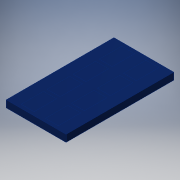
# Autodesk Inventor part: Assembly Plate
Saved by Autodesk Inventor 2019.4 (Build 234330000, 330)
## iProperties
Created: 2021-01-11
Part Number: Assembly Plate
Material: Aluminum, Anodized Blue
Document SubType Name: Modeling
Designer: caleb
Density: 2.7 g/cm^3
Appearance: Anodized - Blue
Author: caleb
Autodesk Inventor part; units mm, degrees
ref_plane "YZ Plane" through (0, 0, 0) normal (1, 0, 0) x (0, 1, 0)
ref_plane "XZ Plane" through (0, 0, 0) normal (0, 1, 0) x (-1, 0, 0)
ref_plane "XY Plane" through (0, 0, 0) normal (0, 0, 1) x (1, 0, 0)
sketch "Sketch1" plane through (0, 0, 0) normal (0, 1, 0) x (-1, 0, 0)
  line L0 (-60, 108) -> (60, 108)
  line L1 (60, 108) -> (60, -108)
  line L2 (60, -108) -> (-60, -108)
  line L3 (-60, -108) -> (-60, 108)
  line L4 (-60, 108) -> (60, -108) construction
  line L5 (60, 108) -> (-60, -108) construction
  point P0 (0, 0)
  dimension "d0" = 120
  dimension "d1" = 216
  constraints: 12 end point, 2 midpoint, 2 parallel, 1 horizontal, 1 perpendicular
  measures "d0" distance of L1.end L2.end
  measures "d1" distance of L0.end L1.end
extrude "Extrusion1" add sketch "Sketch1" along normal blind 14
sketch "Sketch7" plane through (0, 14, 0) normal (0, 1, 0) x (1, 0, 0)
  line L0 (-36.84, -100.8) -> (-11.84, -100.8)
  line L1 (-11.34, -100.3) -> (-11.34, -56.3)
  line L2 (-11.84, -55.8) -> (-36.84, -55.8)
  line L3 (-37.34, -56.3) -> (-37.34, -100.3)
  line L4 (-60, -108) -> (60, -108) projected
  line L5 (-60, 108) -> (-60, -108) projected
  arc A0 (-36.84, -55.8) -> (-37.34, -56.3) centre (-36.84, -56.3) ccw
  arc A1 (-11.34, -56.3) -> (-11.84, -55.8) centre (-11.84, -56.3) ccw
  arc A2 (-11.84, -100.8) -> (-11.34, -100.3) centre (-11.84, -100.3) ccw
  arc A3 (-37.34, -100.3) -> (-36.84, -100.8) centre (-36.84, -100.3) ccw
  arc A4 (-11.84, -48.6) -> (-11.34, -48.1) centre (-11.84, -48.1) ccw
  arc A5 (-37.34, -48.1) -> (-36.84, -48.6) centre (-36.84, -48.1) ccw
  line L6 (-11.34, -48.1) -> (-11.34, -4.1)
  line L7 (-37.34, -4.1) -> (-37.34, -48.1)
  line L8 (-11.84, -3.6) -> (-36.84, -3.6)
  arc A6 (-36.84, -3.6) -> (-37.34, -4.1) centre (-36.84, -4.1) ccw
  arc A7 (-11.34, -4.1) -> (-11.84, -3.6) centre (-11.84, -4.1) ccw
  line L9 (-36.84, -48.6) -> (-11.84, -48.6)
  arc A8 (-11.84, 3.6) -> (-11.34, 4.1) centre (-11.84, 4.1) ccw
  arc A9 (-37.34, 4.1) -> (-36.84, 3.6) centre (-36.84, 4.1) ccw
  line L10 (-11.34, 4.1) -> (-11.34, 48.1)
  line L11 (-37.34, 48.1) -> (-37.34, 4.1)
  line L12 (-11.84, 48.6) -> (-36.84, 48.6)
  arc A10 (-36.84, 48.6) -> (-37.34, 48.1) centre (-36.84, 48.1) ccw
  arc A11 (-11.34, 48.1) -> (-11.84, 48.6) centre (-11.84, 48.1) ccw
  line L13 (-36.84, 3.6) -> (-11.84, 3.6)
  arc A12 (-11.84, 55.8) -> (-11.34, 56.3) centre (-11.84, 56.3) ccw
  arc A13 (-37.34, 56.3) -> (-36.84, 55.8) centre (-36.84, 56.3) ccw
  line L14 (-11.34, 56.3) -> (-11.34, 100.3)
  line L15 (-37.34, 100.3) -> (-37.34, 56.3)
  line L16 (-11.84, 100.8) -> (-36.84, 100.8)
  arc A14 (-36.84, 100.8) -> (-37.34, 100.3) centre (-36.84, 100.3) ccw
  arc A15 (-11.34, 100.3) -> (-11.84, 100.8) centre (-11.84, 100.3) ccw
  line L17 (-36.84, 55.8) -> (-11.84, 55.8)
  arc A16 (36.82, -100.8) -> (37.32, -100.3) centre (36.82, -100.3) ccw
  arc A17 (11.32, -100.3) -> (11.82, -100.8) centre (11.82, -100.3) ccw
  line L18 (37.32, -100.3) -> (37.32, -56.3)
  line L19 (11.32, -56.3) -> (11.32, -100.3)
  line L20 (36.82, -55.8) -> (11.82, -55.8)
  arc A18 (11.82, -55.8) -> (11.32, -56.3) centre (11.82, -56.3) ccw
  arc A19 (37.32, -56.3) -> (36.82, -55.8) centre (36.82, -56.3) ccw
  line L21 (11.82, -100.8) -> (36.82, -100.8)
  arc A20 (36.82, -48.6) -> (37.32, -48.1) centre (36.82, -48.1) ccw
  arc A21 (11.32, -48.1) -> (11.82, -48.6) centre (11.82, -48.1) ccw
  line L22 (37.32, -48.1) -> (37.32, -4.1)
  line L23 (11.32, -4.1) -> (11.32, -48.1)
  line L24 (36.82, -3.6) -> (11.82, -3.6)
  arc A22 (11.82, -3.6) -> (11.32, -4.1) centre (11.82, -4.1) ccw
  arc A23 (37.32, -4.1) -> (36.82, -3.6) centre (36.82, -4.1) ccw
  line L25 (11.82, -48.6) -> (36.82, -48.6)
  arc A24 (36.82, 3.6) -> (37.32, 4.1) centre (36.82, 4.1) ccw
  arc A25 (11.32, 4.1) -> (11.82, 3.6) centre (11.82, 4.1) ccw
  line L26 (37.32, 4.1) -> (37.32, 48.1)
  line L27 (11.32, 48.1) -> (11.32, 4.1)
  line L28 (36.82, 48.6) -> (11.82, 48.6)
  arc A26 (11.82, 48.6) -> (11.32, 48.1) centre (11.82, 48.1) ccw
  arc A27 (37.32, 48.1) -> (36.82, 48.6) centre (36.82, 48.1) ccw
  line L29 (11.82, 3.6) -> (36.82, 3.6)
  arc A28 (36.82, 55.8) -> (37.32, 56.3) centre (36.82, 56.3) ccw
  arc A29 (11.32, 56.3) -> (11.82, 55.8) centre (11.82, 56.3) ccw
  line L30 (37.32, 56.3) -> (37.32, 100.3)
  line L31 (11.32, 100.3) -> (11.32, 56.3)
  line L32 (36.82, 100.8) -> (11.82, 100.8)
  arc A30 (11.82, 100.8) -> (11.32, 100.3) centre (11.82, 100.3) ccw
  arc A31 (37.32, 100.3) -> (36.82, 100.8) centre (36.82, 100.3) ccw
  line L33 (11.82, 55.8) -> (36.82, 55.8)
  point P0 (0, 0)
  point P1 (-37.34, -100.8)
  point P2 (-11.34, -100.8)
  point P3 (-37.34, -55.8)
  point P4 (-37.34, -48.6)
  point P5 (-11.34, -48.6)
  point P6 (-37.34, -3.6)
  point P7 (-37.34, 3.6)
  point P8 (-11.34, 3.6)
  point P9 (-37.34, 48.6)
  point P10 (-37.34, 55.8)
  point P11 (-11.34, 55.8)
  point P12 (-37.34, 100.8)
  point P13 (11.32, -100.8)
  point P14 (37.32, -100.8)
  point P15 (11.32, -55.8)
  point P16 (11.32, -48.6)
  point P17 (37.32, -48.6)
  point P18 (11.32, -3.6)
  point P19 (11.32, 3.6)
  point P20 (37.32, 3.6)
  point P21 (11.32, 48.6)
  point P22 (11.32, 55.8)
  point P23 (37.32, 55.8)
  point P24 (11.32, 100.8)
  dimension "d76" = 45
  dimension "d77" = 26
  dimension "d78" = 7.2
  dimension "d79" = 22.66
  dimension "d80" = 0.5
  dimension "d83" = 52.2
  dimension "d86" = 48.66
  constraints: 64 end point, 64 point on circle, 48 point on line, 32 centre point, 8 tangent, 3 equal radius, 2 horizontal, 2 parallel, 1 perpendicular, 1 vertical, 161 other
  measures "d76" distance of point (-37.34, -55.8) point (-37.34, -100.8)
  measures "d77" distance of point (-37.34, -100.8) point (-11.34, -100.8)
  measures "d78" distance between parallel lines of L4 L0
  measures "d79" distance between parallel lines of L5 L3
  measures "d80" radius of A0
  measures "d83" distance of A2.centre A4.centre
  measures "d86" distance of A2.centre A16.centre
extrude "Extrusion6" cut sketch "Sketch7" against normal blind 0.1
body "Solid1"
